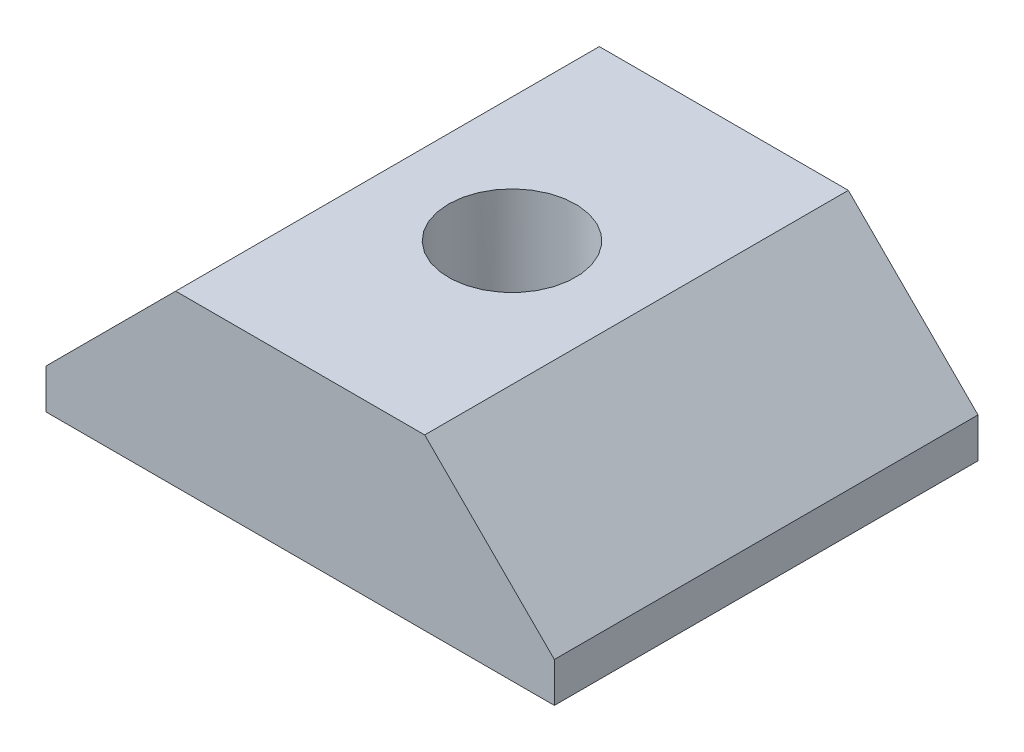
# Autodesk Inventor part: сухарь
Saved by Autodesk Inventor 2024.2 (Build 282272000, 272)
## iProperties
Created: 2026-02-10
Part Number: сухарь
Material: Типовые
Document SubType Name: Modeling
Designer: katya_notebook
Density: 1 g/cm^3
Appearance: По умолчанию
Author: katya_notebook
Autodesk Inventor part; units mm, degrees
ref_plane "YZ Plane" through (0, 0, 0) normal (1, 0, 0) x (0, 1, 0)
ref_plane "XZ Plane" through (0, 0, 0) normal (0, 1, 0) x (-1, 0, 0)
ref_plane "XY Plane" through (0, 0, 0) normal (0, 0, 1) x (1, 0, 0)
ref_plane "РабПлоскость1" through (-175.2223, 354.288, -333.1549) normal (0, 0, -1) x (-1, 0, 0)
sketch "Эскиз1" plane through (-175.2223, 354.288, -333.1549) normal (0, 0, -1) x (-1, 0, 0)
  line L0 (-2.9393, -4) -> (-6, -7.0607) projected
  line L1 (-0.3, -4) -> (-2.9393, -4) projected
  line L2 (2.9393, -4) -> (0.3, -4) projected
  line L3 (6, -7.0607) -> (2.9393, -4) projected
  line L4 (6, -8) -> (6, -7.0607) projected
  line L5 (3, -8) -> (6, -8) projected
  line L6 (-6, -8) -> (-3, -8) projected
  line L7 (-6, -7.0607) -> (-6, -8) projected
  line L8 (0, -3.7) -> (-0.3, -4) projected
  line L9 (0.3, -4) -> (0, -3.7) projected
  line L10 (-2.9393, -4) -> (2.9393, -4)
  line L11 (6, -7.0607) -> (2.9393, -4)
  line L12 (3, -8) -> (6, -8)
  line L13 (6, -8) -> (6, -7.0607)
  line L14 (-3, -8) -> (-6, -8)
  line L15 (-6, -7.0607) -> (-6, -8)
  line L16 (-2.9393, -4) -> (-6, -7.0607)
  line L17 (3, -8) -> (-2.9393, -8)
  line L18 (-2.9393, -8) -> (-3, -8)
  point P0 (-175.2223, -354.288)
  point P1 (0.3, -4)
  constraints: 18 end point, 3 collinear, 3 perpendicular, 1 horizontal, 1 point on line
extrude "Выдавливание1" add sketch "Эскиз1" against normal blind 10 contours L1 L10 L2 L3 L4 L5 L17 L18 L6 L7 L0
sketch "Эскиз2" plane through (-181.2223, 346.288, -333.1549) normal (0, -1, 0) x (1, 0, 0)
  circle A0 centre (6, 26.9999) radius 2 projected
  circle A1 centre (6, 5) radius 1.5
  line L0 (0, 10) -> (12, 10) projected
  point P0 (181.2223, 333.1549)
  dimension "d2" = 3
  dimension "d3" = 5
  constraints: 1 centre point, 1 vertical alignment
  measures "d2" diameter of A1
  measures "d3" distance from line of L0 A1.centre
extrude "Выдавливание2" cut sketch "Эскиз2" against normal blind 10 contours A1
